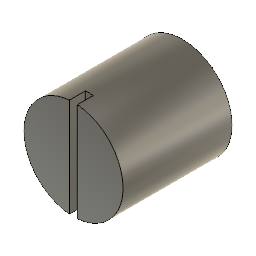
_m10.0842c12e-ae75-486b-aa91-c357400f3b05 (Autodesk Fusion 360 design; units mm, degrees)
Autodesk Fusion 360 part; units mm, degrees
sketch "Sketch1" plane through (0, 0, 0) normal (0, 1, 0) x (1, 0, 0)
  circle A0 centre (0, 0) radius 5
  dimension "d1" = 10
  constraint coincident A0.centre origin
  measures "d1" diameter of A0
extrude "Extrude1" add sketch "Sketch1" along normal blind 11
sketch "Sketch2" plane through (0, 0, 0) normal (1, 0, 0) x (0, 1, 0)
sketch "Sketch3" plane through (0, 0, 0) normal (0, 1, 0) x (1, 0, 0)
  circle A0 centre (0, 0) radius 5
  line L0 (-0.398, -4.9841) -> (-0.398, 4.9841)
  line L1 (0.398, 4.9841) -> (0.398, -4.9841)
  line L2 (-0.398, -4.9841) -> (-0.398, -5.1)
  line L3 (-0.398, -5.1) -> (0.4, -5.1)
  line L4 (0.4, -5.1) -> (0.398, -4.9841)
  line L5 (0.398, 4.9841) -> (0.398, 5.2684)
  line L6 (0.398, 5.2684) -> (-0.5, 5.2684)
  line L7 (-0.5, 5.2684) -> (-0.398, 4.9841)
  constraint coincident A0 L0.start
  constraint coincident A0 L0.end
  constraint vertical L0
  constraint coincident A0 L1.start
  constraint coincident A0 L1.end
  constraint parallel L0 L1
  constraint parallel L0 L2
  constraint perpendicular L2 L3
  constraint parallel L1 L5
  constraint perpendicular L5 L6
extrude "Extrude2" cut sketch "Sketch3" along normal blind 1.6 contours A0 L0 L1 | A0 L5 L6 L7 | A0 L2 L3 L4
